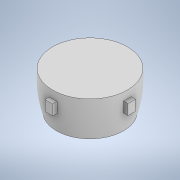
# Autodesk Inventor part: Pommeau globe blanc
Saved by Autodesk Inventor 2021 (Build 250183000, 183)
## iProperties
Created: 2020-09-18
Part Number: Pommeau globe blanc
Material: Générique
Document SubType Name: Modeling
Designer: Utilisateur
Density: 1 g/cm^3
Appearance: Par défaut
Author: Utilisateur
Autodesk Inventor part; units mm, degrees
ref_plane "YZ Plane" through (0, 0, 0) normal (1, 0, 0) x (0, 1, 0)
ref_plane "XZ Plane" through (0, 0, 0) normal (0, 1, 0) x (-1, 0, 0)
ref_plane "XY Plane" through (0, 0, 0) normal (0, 0, 1) x (1, 0, 0)
sketch "Esquisse1" plane through (0, 0, 0) normal (0, 0, 1) x (1, 0, 0)
  circle A0 centre (0, 0) radius 25
  line L0 (0, 28.8291) -> (0, -38.3219)
  line L1 (-31.3088, 0) -> (57.5068, 0)
  arc A1 (22.3616, -25) -> (25, 0) centre (-41.3202, -5.6401) ccw
  line L2 (0, -25) -> (22.3616, -25)
  point P0 (0, 25)
  point P1 (0, -25)
  point P2 (-25, 0)
  constraints: 6 end point, 4 point on circle, 2 centre point, 1 coincident, 1 horizontal, 1 perpendicular, 1 point on line, 1 tangent, 1 vertical
revolve "Révolution1" add sketch "Esquisse1" angle 360 about axis through (0, 28.8291, 0) along (0, -1, 0) picked at (-1.8543, -16.4577) contours A0 L1 L0 | A0 A1 L2
sketch "Esquisse2" plane through (0, 0, 0) normal (1, 0, 0) x (0, 1, 0)
  line L0 (-5, 2.625) -> (-12, 2.625)
  line L1 (-12, 2.625) -> (-12, -2.375)
  line L2 (-12, -2.375) -> (-5, -2.375)
  line L3 (-5, -2.375) -> (-5, 2.625)
  line L4 (-5, 2.625) -> (-12, -2.375) construction
  line L5 (-12, 2.625) -> (-5, -2.375) construction
  line L6 (0, 25) -> (0, -25) projected
  point P0 (0, 0)
  point P1 (-8.5, 0.125)
  dimension "d5" = 7
  dimension "d6" = 5
  dimension "d11" = 5
  constraints: 12 end point, 2 midpoint, 2 parallel, 1 horizontal, 1 perpendicular
  measures "d5" distance of L0.start L0.end
  measures "d6" distance of L2.end L0.start
  measures "d11" distance between parallel lines of L6 L3
extrude "Extrusion1" add sketch "Esquisse2" along normal mid plane 56
sketch "Esquisse3" plane through (0, 0, 0) normal (0, 0, 1) x (1, 0, 0)
  line L0 (-2, -5) -> (3, -5)
  line L1 (3, -5) -> (3, -12)
  line L2 (3, -12) -> (-2, -12)
  line L3 (-2, -12) -> (-2, -5)
  line L4 (-2, -5) -> (3, -12) construction
  line L5 (3, -5) -> (-2, -12) construction
  line L6 (-25, 0) -> (25, 0) projected
  point P0 (0, 0)
  point P1 (0.5, -8.5)
  dimension "d12" = 7
  dimension "d13" = 5
  dimension "d14" = 5
  constraints: 12 end point, 2 midpoint, 2 parallel, 1 horizontal, 1 perpendicular
  measures "d12" distance of L2.end L0.start
  measures "d13" distance of L1.end L2.end
  measures "d14" distance between parallel lines of L6 L0
extrude "Extrusion2" add sketch "Esquisse3" along normal mid plane 56
